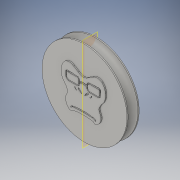
# Autodesk Inventor part: winston_wheels
Saved by Autodesk Inventor 2016 (Build 200138000, 138)
## iProperties
Created: 2017-09-05
Part Number: winston_wheels
Material: Generic
Document SubType Name: Modeling
Designer: Student
Density: 1 g/cm^3
Appearance: Default
Author: Student
Autodesk Inventor part; units mm, degrees
ref_plane "XZ Plane" through (0, 0, 0) normal (0, 1, 0) x (-1, 0, 0)
ref_plane "XY Plane" through (0, 0, 0) normal (0, 0, 1) x (1, 0, 0)
sketch "Sketch1" plane through (0, 0, 0) normal (0, 0, 1) x (1, 0, 0)
  circle A0 centre (0, 0) radius 21.971
  dimension "d0" = 43.942
  constraints: 1 centre point, 1 coincident
  measures "d0" diameter of A0
extrude "Extrusion1" add sketch "Sketch1" along normal blind 6.35
sketch "Sketch3" plane through (0, 0, 0) normal (1, 0, 0) x (0, 1, 0)
  line L0 (21.971, 0) -> (21.971, 6.35) projected
  circle A0 centre (21.971, 3.175) radius 2.54
  line L1 (0, -1.27) -> (0, 7.62) projected
  point P0 (0, 0)
  dimension "d37" = 5.08
  constraints: 1 centre point, 1 midpoint
  measures "d37" diameter of A0
revolve "Revolution1" cut sketch "Sketch3" angle 360 about axis through (0, 0, -10) along (0, 0, 1)
sketch "Sketch4" plane through (0, 0, 0) normal (0, 0, -1) x (-1, 0, 0)
  line L0 (2.4384, -2.5883) -> (2.4384, 2.5883)
  line L1 (-2.4384, -2.5883) -> (-2.4384, 2.5883)
  arc A0 (2.4384, 2.5883) -> (-2.4384, 2.5883) centre (0, 0) ccw
  arc A1 (-2.4384, -2.5883) -> (2.4384, -2.5883) centre (0, 0) ccw
  dimension "d44" = 4.8768
  dimension "d45" = 3.556
  dimension "d46" = 5.1766
  dimension "d47" = 2.4384
  constraints: 4 end point, 4 point on circle, 2 centre point, 1 coincident, 1 parallel, 1 vertical
  measures "d44" distance between parallel lines of L1 L0
  measures "d45" radius of A0
  measures "d46" distance of L0.start L0.end
  measures "d47" distance from line of point (0, 0) L0
extrude "Extrusion3" cut sketch "Sketch4" against normal blind 5.2324
sketch "Sketch6" plane through (0, 0, 6.35) normal (0, 0, 1) x (1, 0, 0)
  line L0 (-7.9781, 5.9587) -> (-3.1219, 5.9587)
  line L1 (-2.4432, 5.408) -> (-2.4432, 3.3347)
  line L2 (-3.0554, 2.6517) -> (-7.4903, 2.6517)
  line L3 (-8.5392, 3.4123) -> (-8.5392, 5.408)
  line L4 (8.1395, 5.9587) -> (3.0702, 5.9587)
  line L5 (2.4177, 5.1909) -> (2.4177, 3.3347)
  line L6 (3.141, 2.6517) -> (7.6368, 2.6517)
  line L7 (8.3543, 3.4828) -> (8.3543, 5.7492)
  arc A0 (-7.9781, 5.9587) -> (-8.5392, 5.408) centre (-7.8712, 5.2886) ccw
  arc A1 (-2.4432, 5.408) -> (-3.1219, 5.9587) centre (-3.4653, 4.8418) ccw
  arc A2 (-3.0554, 2.6517) -> (-2.4432, 3.3347) centre (-3.5014, 3.6673) ccw
  arc A3 (-8.5392, 3.4123) -> (-7.4903, 2.6517) centre (-6.8939, 4.5778) ccw
  arc A4 (3.0702, 5.9587) -> (2.4177, 5.1909) centre (3.5383, 4.8998) ccw
  arc A5 (8.3543, 5.6495) -> (8.0528, 5.9587) centre (8.0962, 5.6994) ccw
  arc A6 (7.6368, 2.6517) -> (8.3543, 3.4828) centre (7.3237, 3.6474) ccw
  arc A7 (2.4177, 3.3347) -> (3.141, 2.6517) centre (3.4866, 3.7422) ccw
  line L8 (-2.8273, 2.181) -> (-7.8294, 2.181)
  line L9 (-9.066, 4.1804) -> (-9.066, 5.8577)
  arc A8 (-8.3112, 6.6529) -> (-9.066, 5.8577) centre (-8.0508, 5.6499) ccw
  arc A9 (-1.8603, 5.1686) -> (-2.5407, 6.3223) centre (-4.0116, 4.6774) ccw
  arc A10 (-8.9398, 3.1929) -> (-7.8294, 2.181) centre (-6.9951, 4.2118) ccw
  arc A11 (-2.8273, 2.181) -> (-1.8603, 3.1929) centre (-3.6789, 3.9629) ccw
  line L10 (-9.066, 4.1804) -> (-8.9398, 3.1929)
  line L11 (-6.2315, 6.6529) -> (-2.5407, 6.3223)
  line L12 (-8.3112, 6.6529) -> (-6.2315, 6.6529)
  line L13 (2.9922, 2.181) -> (7.8619, 2.181)
  arc A12 (3.1111, 6.4373) -> (1.9198, 5.2197) centre (3.1377, 5.2197) ccw
  arc A13 (9.0645, 5.9957) -> (8.0528, 6.7425) centre (7.5959, 5.0648) ccw
  arc A14 (7.8619, 2.181) -> (8.9541, 3.0279) centre (6.8209, 4.6512) ccw
  arc A15 (1.9198, 3.1929) -> (2.9922, 2.181) centre (4.2129, 4.5489) ccw
  line L14 (3.1111, 6.4373) -> (8.0528, 6.7425)
  line L15 (9.0645, 5.9957) -> (8.9541, 3.0279)
  arc A16 (1.9198, 4.8418) -> (-1.8603, 4.9163) centre (-0.1121, -2.322) ccw
  arc A17 (1.9198, 3.786) -> (-1.8603, 3.8303) centre (-0.0039, 0.936) ccw
  line L16 (-1.8603, 5.1686) -> (-1.8603, 4.9163)
  line L17 (-1.8603, 3.8303) -> (-1.8603, 3.1929)
  line L18 (1.9198, 5.2197) -> (1.9198, 4.8418)
  line L19 (1.9198, 3.786) -> (1.9198, 3.1929)
  arc A18 (-4.1357, 0.9038) -> (-4.464, 0.8903) centre (-4.3032, 0.9784) ccw
  arc A19 (-4.1357, 0.9038) -> (-3.3316, -0.031) centre (-2.8724, 1.1772) ccw
  arc A20 (-4.464, 0.8903) -> (-3.3818, -0.1148) centre (-3.2049, 1.1609) ccw
  arc A21 (-3.3818, -0.1148) -> (-3.3316, -0.031) centre (-3.4365, -0.0251) ccw
  arc A22 (-2.1108, 1.4905) -> (-2.6145, 0.9784) centre (-2.3487, 1.2208) ccw
  arc A23 (-2.6145, 0.9784) -> (-0.6722, -0.4025) centre (3.6836, 7.7805) ccw
  arc A24 (-0.6722, -0.4025) -> (-2.1108, 1.4905) centre (-6.6731, -3.4698) ccw
  arc A25 (2.5831, 0.8903) -> (2.0688, 1.473) centre (2.3523, 1.2049) ccw
  arc A26 (2.0688, 1.473) -> (0.6026, -0.4845) centre (7.4607, -4.0937) ccw
  arc A27 (0.6026, -0.4845) -> (2.5831, 0.8903) centre (-6.0361, 11.1925) ccw
  arc A28 (4.464, 0.8903) -> (4.1357, 0.9038) centre (4.3032, 0.9784) ccw
  arc A29 (3.3316, -0.031) -> (4.1357, 0.9038) centre (2.8724, 1.1772) ccw
  arc A30 (3.3818, -0.1148) -> (4.464, 0.8903) centre (3.2049, 1.1609) ccw
  arc A31 (3.3316, -0.031) -> (3.3818, -0.1148) centre (3.4365, -0.0251) ccw
  arc A32 (-10.4825, 8.7498) -> (-10.9959, 2.4175) centre (-4.4773, 5.076) ccw
  arc A33 (-4.9108, 9.9288) -> (-10.4825, 8.7498) centre (-7.248, 7.2189) ccw
  arc A34 (-2.6544, 8.5138) -> (-4.9108, 9.9288) centre (-11.9242, -3.7622) ccw
  arc A35 (-2.6544, 8.5138) -> (0.0366, 7.495) centre (0.4309, 12.5996) ccw
  arc A36 (0.0366, 7.495) -> (2.6448, 8.5138) centre (-0.3941, 12.4455) ccw
  arc A37 (4.8823, 9.9288) -> (2.6448, 8.5138) centre (8.9507, 1.0186) ccw
  arc A38 (9.6553, 9.9288) -> (4.8823, 9.9288) centre (7.2688, 6.9719) ccw
  arc A39 (11.4395, 5.9587) -> (9.6553, 9.9288) centre (5.3948, 5.6281) ccw
  line L20 (11.4395, 5.9587) -> (11.4395, 3.9629)
  arc A40 (9.3566, -0.1148) -> (11.4395, 3.9629) centre (5.3141, 4.521) ccw
  arc A41 (9.3566, -0.1148) -> (8.2844, -2.0877) centre (249.5341, -131.9234) ccw
  arc A42 (8.2844, -2.0877) -> (8.2844, -3.7622) centre (10.1594, -2.9249) ccw
  arc A43 (9.1939, -6.1968) -> (8.2844, -3.7622) centre (-25.3645, -17.7196) ccw
  arc A44 (6.5358, -10.6449) -> (9.1939, -6.1968) centre (4.4751, -6.3952) ccw
  arc A45 (5.3141, -9.9262) -> (6.5358, -10.6449) centre (6.59, -9.1552) ccw
  arc A46 (5.3141, -9.9262) -> (-5.3283, -9.9262) centre (-0.0071, -38.9072) ccw
  arc A47 (-7.7165, -9.9262) -> (-5.3283, -9.9262) centre (-6.5224, -9.3094) ccw
  arc A48 (-8.7449, -8.4473) -> (-7.7165, -9.9262) centre (-4.8079, -6.8067) ccw
  arc A49 (-8.2225, -3.6148) -> (-8.7449, -8.4473) centre (-4.0871, -6.5063) ccw
  line L21 (-8.2225, -3.6148) -> (-8.2225, -2.322)
  arc A50 (-10.9959, 2.4175) -> (-9.5717, 0.2172) centre (-4.4773, 5.076) ccw
  arc A51 (-8.2225, -2.322) -> (-9.5717, 0.2172) centre (-13.1177, -3.295) ccw
  arc A52 (-6.6046, -8.895) -> (-6.0361, -8.9081) centre (-6.32, -8.8845) ccw
  arc A53 (-5.4148, -8.1105) -> (-6.6046, -8.895) centre (-5.2651, -9.632) ccw
  arc A54 (-0.0071, -7.6136) -> (-5.4148, -8.1105) centre (-0.7065, -29.6779) ccw
  arc A55 (-4.5479, -8.3999) -> (-6.0361, -8.9081) centre (-4.6931, -10.4079) ccw
  arc A56 (-0.0071, -8.2137) -> (-4.5479, -8.3999) centre (-0.3573, -55.1276) ccw
  line L22 (-0.0039, 0.936) -> (-0.0039, -3.295)
  arc A57 (6.0284, -8.9081) -> (6.5969, -8.895) centre (6.3123, -8.8845) ccw
  arc A58 (6.5969, -8.895) -> (5.4071, -8.1105) centre (5.2574, -9.632) ccw
  arc A59 (5.4071, -8.1105) -> (-0.0006, -7.6136) centre (0.6988, -29.6779) ccw
  arc A60 (6.0284, -8.9081) -> (4.5402, -8.3999) centre (4.6854, -10.4079) ccw
  arc A61 (4.5402, -8.3999) -> (-0.0006, -8.2137) centre (0.3496, -55.1276) ccw
  line L23 (-0.0071, -7.6136) -> (-0.0006, -7.6136)
  line L24 (-0.0071, -8.2137) -> (-0.0006, -8.2137)
  point P0 (0, 0)
  point P1 (6.5147, -9.3094)
  point P2 (4.8002, -6.8067)
  point P3 (4.0794, -6.5063)
  constraints: 126 point on circle, 62 centre point, 50 end point, 14 symmetric about line, 8 parallel, 4 horizontal, 4 perpendicular, 4 tangent, 2 point on line, 2 vertical, 5 other
extrude "Extrusion4" add sketch "Sketch6" along normal blind 0.635 contours L0 A1 L1 A2 L2 A3 L3 A0 | A5 L7 A6 L6 A7 L5 A4 L4 | A33 A34 A35 A36 A37 A38 A39 L20 A40 A41 A42 A43 A44 A45 A46 A47 A48 A49 L21 A51 A50 A32
body "Solid1"
